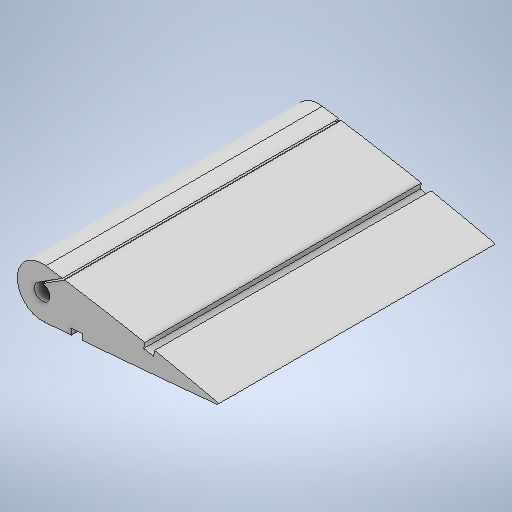
# Autodesk Inventor part: 2P.03.01.02.IM.AileronBody
Saved by Autodesk Inventor 2025.2 (Build 292293000, 293)
## iProperties
Created: 2024-12-30
Part Number: 2P.03.01.02.IM.AileronBody
Material: Generic
Document SubType Name: Modeling
Designer: Imist
Density: 1 g/cm^3
Appearance: Default
Author: Imist
Autodesk Inventor part; units mm, degrees
ref_plane "YZ Plane" through (0, 0, 0) normal (1, 0, 0) x (0, 1, 0)
ref_plane "XZ Plane" through (0, 0, 0) normal (0, 1, 0) x (-1, 0, 0)
ref_plane "XY Plane" through (0, 0, 0) normal (0, 0, 1) x (1, 0, 0)
sketch "Sketch1" plane through (0, 0, 0) normal (0, 0, 1) x (1, 0, 0)
  line L0 (14.8631, 7.5798) -> (15.4426, 10.5233)
  line L1 (19.8631, 6.5954) -> (14.8631, 7.5798)
  line L2 (20.4426, 9.5389) -> (19.8631, 6.5954)
  line L3 (15.4426, 10.5233) -> (20.4426, 9.5389)
  spline S0 degree 2 poles (-23.8666, 11.2126) (-23.7579, 11.1965) (-23.6493, 11.1804) knots 0 0 0 1 1 1
  line L4 (-23.6714, 11.1837) -> (-23.6271, 11.1771) construction
  arc A0 (-23.6315, 11.1777) -> (-23.667, 11.183) centre (-39.2289, -93.6435) ccw construction
  line L5 (-16.6401, -4.573) -> (-16.8877, -1.5832)
  line L6 (-16.8877, -1.5832) -> (-22.5535, -2.0523)
  line L7 (-22.5535, -2.0523) -> (-22.306, -5.0421)
  line L8 (-22.306, -5.0421) -> (-16.6401, -4.573)
  arc A1 (-35.4368, 19.2227) -> (-36.2948, -6.1813) centre (-37.3325, 6.5703) ccw
  arc A2 (-39.4856, 9.9414) -> (-37.0323, 10.559) centre (-37.3325, 6.5703) ccw
  arc A3 (-3.2063, -3.4382) -> (-3.985, -3.5046) centre (-2.8932, -11.7051) ccw
  line L9 (-18.6283, -4.7387) -> (-14.6519, -4.4072) construction
  arc A4 (-15.0495, -4.4405) -> (-18.2307, -4.7057) centre (808.5789, -9970.4655) ccw construction
  spline S1 degree 4 poles (-36.2948, -6.1813) (-30.5718, -5.7155) (-22.3369, -5.0486) (-20.2521, -4.874) (-16.6401, -4.573) knots 0 0 0 0 0 1 1 1 1 1
  line L10 (-3.2856, -3.445) -> (-3.1269, -3.4314) construction
  arc A5 (-3.2697, -3.4436) -> (-3.1428, -3.4328) centre (-407.6993, 4735.9123) ccw construction
  spline S2 degree 2 poles (-3.985, -3.5046) (-3.5952, -3.4714) (-3.2063, -3.4382) knots 0 0 0 1 1 1
  spline S3 degree 4 poles (13.7634, -1.9753) (14.2602, -1.9317) (14.4328, -1.9172) (27.2695, -0.78) (31.7218, -0.3887) (39.3561, 0.3576) (45.9817, 0.8441) (50.2399, 1.5266) (52.6989, 1.2631) (53.123, 2.0529) knots 0 0 0 0 0 0.172623 0.316544 0.485874 0.63811 0.76971 1 1 1 1 1
  line L11 (9.1543, -2.3795) -> (18.3725, -1.5711) construction
  arc A6 (17.4512, -1.6584) -> (10.0767, -2.3052) centre (105.4782, -1047.7355) ccw construction
  line L12 (-22.306, -5.0421) -> (-16.6401, -4.573) construction
  line L13 (-16.6401, -4.573) -> (-9.1202, -3.9503) construction
  line L14 (-9.1202, -3.9503) -> (3.1193, -2.9368) construction
  line L15 (3.1193, -2.9368) -> (14.267, -1.9311) construction
  spline S4 degree 4 poles (-22.306, -5.0421) (-16.6401, -4.573) (-9.1202, -3.9503) (3.1193, -2.9368) (14.267, -1.9311) knots 1 1 1 1 1 2 2 2 2 2
  line L16 (-26.9697, 17.935) -> (-39.4856, 9.9414)
  spline S5 degree 3 poles (-35.4368, 19.2227) (-32.6135, 18.7997) (-29.7852, 18.3714) (-26.9697, 17.935) knots 0 0 0 0 1 1 1 1
  spline S6 degree 4 poles (-25.7746, 17.7483) (-23.5566, 17.4023) (-21.2363, 17.0457) (-7.1409, 14.7244) (3.1994, 12.8429) (14.4252, 10.7509) (24.006, 8.8301) (32.5032, 7.1028) (39.4707, 5.5402) (46.2845, 4.1673) (50.3, 2.9609) (52.8188, 2.8949) (53.123, 2.0529) knots 0 0 0 0 0 0.150419 0.261394 0.381802 0.49599 0.602914 0.70135 0.789818 0.86627 1 1 1 1 1
  line L17 (-27.8314, 18.0686) -> (-26.108, 17.8015) construction
  arc A7 (-26.2805, 17.8271) -> (-27.6591, 18.0417) centre (-215.1303, -1196.0826) ccw construction
  line L18 (-26.4936, 17.2899) -> (-37.0323, 10.559)
  line L19 (-26.4936, 17.2899) -> (-25.7746, 17.7483)
  line L20 (-34.0391, 19.0376) -> (-17.51, 16.4591) construction
  arc A8 (-19.1659, 16.6985) -> (-32.389, 18.7613) centre (-210.9554, -1169.3442) ccw construction
  point P0 (0, 0)
  point P1 (17.1316, -7.3867)
  point P2 (-0.812, 3.0577)
  point P3 (53.123, 2.0529)
  point P4 (3.869, 12.7089)
  point P5 (14.924, 10.6239)
  point P6 (24.749, 8.6739)
  point P7 (33.239, 6.9129)
  point P8 (40.31, 5.3889)
  point P9 (45.884, 4.1529)
  point P10 (49.91, 3.2409)
  point P11 (52.34, 2.6829)
  point P12 (-9.1202, -3.9503)
  point P13 (3.1193, -2.9368)
  point P14 (32.813, -0.2751)
  point P15 (40.001, 0.3819)
  point P16 (45.677, 0.9099)
  point P17 (49.781, 1.2969)
  point P18 (52.262, 1.5339)
  point P19 (-50.1188, 7.0059)
  point P20 (53.123, 2.4939)
  point P21 (-50.119, 21.2889)
  point P22 (-50.929, -7.3431)
  point P23 (53.123, 1.6119)
  point P24 (-35.437, 6.5548)
  point P25 (-21.448, 6.0472)
  point P26 (-8.296, 5.5021)
  point P27 (3.869, 4.9385)
  point P28 (14.924, 4.3755)
  point P29 (24.749, 3.8355)
  point P30 (33.239, 3.3384)
  point P31 (40.31, 2.8998)
  point P32 (45.884, 2.5411)
  point P33 (49.91, 2.2751)
  point P34 (52.34, 2.1119)
  point P35 (-24.2098, 1.051)
  point P36 (11.5574, 4.345)
  point P37 (-18.271, 10.3498)
  point P38 (-13.0102, 9.4738)
  point P39 (-8.1442, 8.6074)
  point P40 (-3.7222, 7.7734)
  point P41 (0.2078, 6.9934)
  point P42 (3.6038, 6.289)
  point P43 (6.4322, 5.6794)
  point P44 (8.6618, 5.185)
  point P45 (10.2722, 4.8202)
  point P46 (11.2442, 4.597)
  point P47 (-18.6142, 1.507)
  point P48 (-13.3402, 1.9474)
  point P49 (-8.4454, 2.365)
  point P50 (-3.985, 2.7514)
  point P51 (-0.0106, 3.103)
  point P52 (3.4334, 3.4138)
  point P53 (6.3086, 3.6766)
  point P54 (8.579, 3.8878)
  point P55 (10.2206, 4.0426)
  point P56 (11.213, 4.1374)
  point P57 (13.7634, -1.9753)
  point P58 (-26.5962, 17.8762)
  point P59 (-16.6401, -4.5728)
  dimension "d0" = 3
  dimension "d1" = 5
  dimension "d2" = 52.7751
  dimension "d3" = 3
  dimension "d4" = 5.6658
  dimension "d5" = 8
  dimension "d10" = 0.8
  constraints: 34 end point, 13 point on circle, 12 midpoint, 9 centre point, 4 coincident, 4 parallel, 2 perpendicular, 2 tangent, 1 point on line, 49 other
  measures "d0" distance of L2.start L1.start
  measures "d1" horizontal distance of L2.start L0.end
  measures "d2" horizontal distance of A1.centre L0.end
  measures "d3" distance of L5.end L5.start
  measures "d4" horizontal distance of L5.end L6.end
  measures "d5" diameter of A2
  measures "d10" distance between parallel lines of L16 L18
extrude "Extrusion2" add sketch "Sketch1" along normal blind 142 contours L1 L2 S6 S3 S4 L5 L6 L7 S1 A1 S5 L16 A2 L18 L19 L0
body "Solid2"
